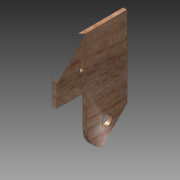
# Autodesk Inventor part: houder
Saved by Autodesk Inventor 2015 (Build 190159000, 159)
## iProperties
Created: 2015-12-31
Part Number: houder
Material: Generic
Document SubType Name: Modeling
Designer: david
Density: 1 g/cm^3
Appearance: Birch - Natural Polished
Author: david
Autodesk Inventor part; units mm, degrees
ref_plane "YZ Plane" through (0, 0, 0) normal (1, 0, 0) x (0, 1, 0)
ref_plane "XZ Plane" through (0, 0, 0) normal (0, 1, 0) x (-1, 0, 0)
ref_plane "XY Plane" through (0, 0, 0) normal (0, 0, 1) x (1, 0, 0)
sketch "Sketch1" plane through (0, 0, 0) normal (1, 0, 0) x (0, 1, 0)
  line L0 (-20, -30) -> (20, -30)
  line L1 (20, -30) -> (20, 30)
  line L2 (20, 30) -> (-20, 30)
  line L3 (-20, 30) -> (-20, -30)
  line L4 (-20, -30) -> (20, 30) construction
  line L5 (20, -30) -> (-20, 30) construction
  circle A0 centre (0, -30) radius 20
  point P0 (0, 0)
  dimension "d0" = 40
  dimension "d1" = 60
  constraints: 12 end point, 3 midpoint, 2 parallel, 1 horizontal, 1 horizontal alignment, 1 perpendicular, 2 other
  measures "d0" distance of L2.end L1.end
  measures "d1" distance of L1.end L0.end
extrude "Extrusion1" add sketch "Sketch1" along normal blind 4
sketch "Sketch4" plane through (4, 0, 0) normal (1, 0, 0) x (0, 0, -1)
  line L0 (-5, 20) -> (-55, 20)
  line L1 (-55, 20) -> (-55, -50)
  line L2 (-55, -50) -> (-5, -50)
  line L3 (-5, -50) -> (-5, 20)
  line L4 (-5, -104.205) -> (-5, 91.5035)
  line L5 (0, -143.3467) -> (0, 130.6452) projected
  dimension "d40" = 50
  dimension "d41" = 70
  dimension "d49" = 5
  dimension "d50" = 0
  constraints: 10 end point, 2 parallel, 1 horizontal, 1 perpendicular, 1 vertical
  measures "d40" distance of L2.end L1.end
  measures "d41" distance of L1.end L0.end
  measures "d49" distance between parallel lines of L5 L4
  measures "d50" distance between parallel lines of L4 L3
extrude "Extrusion4" add sketch "Sketch4" against normal blind 4
sketch "Sketch5" plane through (0, 0, 0) normal (-1, 0, 0) x (0, 0, 1)
  line L0 (34.5, -27) -> (24.2, -27)
  line L1 (24.2, -27) -> (24.2, -22.7)
  line L2 (24.2, -22.7) -> (34.5, -22.7)
  line L3 (34.5, -22.7) -> (34.5, -27)
  line L4 (55, -50) -> (55, -6.689)
  line L5 (55, -50) -> (55, 20) projected
  line L6 (55, -50) -> (10.2215, -50)
  line L7 (5, -50) -> (55, -50) projected
  point P0 (55, 20)
  point P1 (20, -20)
  dimension "d20" = 10.3
  dimension "d21" = 4.3
  constraints: 12 end point, 2 parallel, 1 horizontal, 1 perpendicular, 1 point on line, 2 other
  measures "d20" distance of L1.end L2.end
  measures "d21" distance of L0.end L1.end
extrude "Extrusion5" cut sketch "Sketch5" against normal blind 4
sketch "Sketch2" plane through (0, 0, 0) normal (-1, 0, 0) x (0, 0, 1)
  arc A0 (-30, 20) -> (-30, -20) centre (-30, 0) ccw projected
  circle A1 centre (-30, 0) radius 5.15
  point P0 (0, 0)
  dimension "d4" = 10.3
  constraints: 1 centre point, 1 coincident
  measures "d4" diameter of A1
extrude "Extrusion2" cut sketch "Sketch2" against normal blind 4
fillet "Fillet3" radius 15 2 edges at (2, -20, 5) (2, -50, 5)
body "Solid1"
